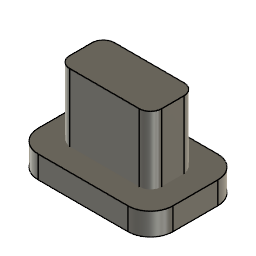
Pulse_button (Autodesk Fusion 360 design; units mm, degrees)
part number: 2026-08-25-02-05-47-490
Autodesk Fusion 360 part; units mm, degrees
sketch "草图1" plane through (0, 0, 0) normal (0, 0, 1) x (1, 0, 0)
  line L0 (1, 0) -> (5, 0)
  line L1 (6, 1) -> (6, 3)
  line L2 (5, 4) -> (1, 4)
  line L3 (0, 3) -> (0, 1)
  arc A0 (1, 4) -> (0, 3) centre (1, 3) ccw
  arc A1 (6, 3) -> (5, 4) centre (5, 3) ccw
  arc A2 (0, 1) -> (1, 0) centre (1, 1) ccw
  arc A3 (5, 0) -> (6, 1) centre (5, 1) ccw
  point P0 (6, 0)
  point P1 (0, 4)
  dimension "d1" = 6
  dimension "d2" = 4
  dimension "d3" = 1
  dimension "d4" = 1
  dimension "d5" = 1
  dimension "d6" = 1
  constraint horizontal L0
  constraint vertical L1
  constraint horizontal L2
  constraint vertical L3
  constraint coincident P1 L2
  constraint coincident P1 L3
  constraint tangent L2 A0
  constraint tangent L3 A0
  constraint tangent L1 A1
  constraint tangent L2 A1
  constraint coincident origin L0
  constraint coincident origin L3
  constraint tangent L0 A2
  constraint tangent L3 A2
  constraint coincident P0 L0
  constraint coincident P0 L1
  constraint tangent L0 A3
  constraint tangent L1 A3
  measures "d1" distance of origin P0
  measures "d2" distance of origin P1
  measures "d3" radius of A0
  measures "d4" radius of A1
  measures "d5" radius of A2
  measures "d6" radius of A3
extrude "拉伸1" add sketch "草图1" along normal blind 1 makes body 1
sketch "草图2" plane through (0, 0, 0) normal (0, 0, 1) x (1, 0, 0)
  line L0 (1.4, 1) -> (4.5, 1)
  line L1 (5, 1.5) -> (5, 2.5)
  line L2 (4.5, 3) -> (1.4, 3)
  line L3 (0.9, 2.5) -> (0.9, 1.5)
  arc A0 (1.4, 3) -> (0.9, 2.5) centre (1.4, 2.5) ccw
  arc A1 (5, 2.5) -> (4.5, 3) centre (4.5, 2.5) ccw
  arc A2 (0.9, 1.5) -> (1.4, 1) centre (1.4, 1.5) ccw
  arc A3 (4.5, 1) -> (5, 1.5) centre (4.5, 1.5) ccw
  dimension "d9" = 0.5
  dimension "d10" = 0.5
  dimension "d11" = 0.5
  dimension "d12" = 0.5
  constraint horizontal L0
  constraint vertical L1
  constraint horizontal L2
  constraint vertical L3
  constraint tangent L2 A0
  constraint tangent L3 A0
  constraint tangent L1 A1
  constraint tangent L2 A1
  constraint tangent L0 A2
  constraint tangent L3 A2
  constraint tangent L0 A3
  constraint tangent L1 A3
  measures "d9" radius of A0
  measures "d10" radius of A1
  measures "d11" radius of A2
  measures "d12" radius of A3
extrude "拉伸2" add sketch "草图2" along normal blind 4 separate body makes body 2
extrude "拉伸3" cut sketch "草图2" along normal blind 0.5 bodies 1 2
